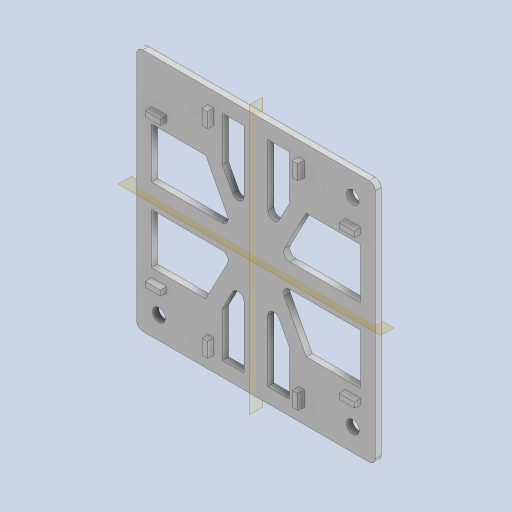
# Autodesk Inventor part: BLTouch-Leveling-Plate_V2
Saved by Autodesk Inventor 2023.2 (Build 272271000, 271)
## iProperties
Created: 2024-02-15
Part Number: BLTouch-Leveling-Plate_V2
Material: Generisch
Document SubType Name: Modeling
Designer: Nils Bade
Density: 1 g/cm^3
Appearance: Vorgabe
Description: Dummy
Auf Bestellliste: True
Author: Nils Bade
Autodesk Inventor part; units mm, degrees
ref_plane "XY Plane" through (0, 0, 0) normal (0, 0, 1) x (1, 0, 0)
sketch "S-Basis" plane through (0, 0, 0) normal (0, 0, 1) x (1, 0, 0)
  line L0 (0, 57.19) -> (0, -57.19) construction
  line L1 (-56, 0) -> (56, 0) construction
  line L2 (-40, 40.85) -> (40, 40.85)
  line L3 (40, 40.85) -> (40, -40.85)
  line L4 (40, -40.85) -> (-40, -40.85)
  line L5 (-40, -40.85) -> (-40, 40.85)
  line L6 (-40, 40.85) -> (40, -40.85) construction
  line L7 (40, 40.85) -> (-40, -40.85) construction
  line L8 (-40, 33.35) -> (40, 33.35) construction
  line L9 (-40, 13.03) -> (40, 13.03) construction
  circle A0 centre (32.5, 33.35) radius 2.15
  circle A1 centre (-32.5, -33.35) radius 2.15
  circle A2 centre (32.5, -33.35) radius 2.15
  line L10 (-40, -40.85) -> (-16.2, -40.85) construction
  line L11 (-16.2, -40.85) -> (-16.2, -25.85) construction
  line L12 (-16.2, -25.85) -> (-40, -25.85) construction
  line L13 (-40, -25.85) -> (-40, -40.85) construction
  line L14 (-40, 40.85) -> (-16.2, 40.85) construction
  line L15 (-16.2, 40.85) -> (-16.2, 25.85) construction
  line L16 (-16.2, 25.85) -> (-40, 25.85) construction
  line L17 (-40, 25.85) -> (-40, 40.85) construction
  line L18 (40, -40.85) -> (16.2, -40.85) construction
  line L19 (16.2, -40.85) -> (16.2, -25.85) construction
  line L20 (16.2, -25.85) -> (40, -25.85) construction
  line L21 (40, -25.85) -> (40, -40.85) construction
  line L22 (40, 40.85) -> (16.2, 40.85) construction
  line L23 (40, 25.85) -> (40, 40.85) construction
  line L24 (16.2, 25.85) -> (40, 25.85) construction
  line L25 (16.2, 40.85) -> (16.2, 25.85) construction
  line L26 (-16.2, -35.85) -> (-14.2, -35.85)
  line L27 (-14.2, -35.85) -> (-14.2, -30.85)
  line L28 (-14.2, -30.85) -> (-16.2, -30.85)
  line L29 (-16.2, -30.85) -> (-16.2, -35.85)
  line L30 (-35, -25.85) -> (-30, -25.85)
  line L31 (-30, -25.85) -> (-30, -23.85)
  line L32 (-30, -23.85) -> (-35, -23.85)
  line L33 (-35, -23.85) -> (-35, -25.85)
  line L34 (-16.2, 35.85) -> (-14.2, 35.85)
  line L35 (-14.2, 35.85) -> (-14.2, 30.85)
  line L36 (-14.2, 30.85) -> (-16.2, 30.85)
  line L37 (-16.2, 30.85) -> (-16.2, 35.85)
  line L38 (-35, 25.85) -> (-30, 25.85)
  line L39 (-30, 25.85) -> (-30, 23.85)
  line L40 (-30, 23.85) -> (-35, 23.85)
  line L41 (-35, 23.85) -> (-35, 25.85)
  line L42 (16.2, -35.85) -> (14.2, -35.85)
  line L43 (14.2, -35.85) -> (14.2, -30.85)
  line L44 (14.2, -30.85) -> (16.2, -30.85)
  line L45 (16.2, -30.85) -> (16.2, -35.85)
  line L46 (35, -25.85) -> (30, -25.85)
  line L47 (30, -25.85) -> (30, -23.85)
  line L48 (30, -23.85) -> (35, -23.85)
  line L49 (35, -23.85) -> (35, -25.85)
  line L50 (14.2, 30.85) -> (16.2, 30.85)
  line L51 (14.2, 35.85) -> (14.2, 30.85)
  line L52 (16.2, 35.85) -> (14.2, 35.85)
  line L53 (16.2, 30.85) -> (16.2, 35.85)
  line L54 (30, 25.85) -> (30, 23.85)
  line L55 (30, 23.85) -> (35, 23.85)
  line L56 (35, 23.85) -> (35, 25.85)
  line L57 (35, 25.85) -> (30, 25.85)
  circle A3 centre (-32.5, 33.35) radius 2.15
  point P0 (-16.2, -33.35)
  point P1 (-16.2, 33.35)
  point P2 (16.2, -33.35)
  point P3 (16.2, 33.35)
  dimension "d0" = 81.7
  dimension "d1" = 80
  dimension "d9" = 4.3
  dimension "d10" = 32.5
  dimension "d11" = 7.5
  dimension "d26" = 15
  dimension "d27" = 23.8
  dimension "d30" = 5
  dimension "d31" = 5
  dimension "d32" = 5
  dimension "d33" = 2
  dimension "d34" = 2
  constraints: 112 end point, 38 symmetric about line, 8 parallel, 6 perpendicular, 6 point on line, 4 centre point, 4 horizontal, 2 midpoint, 2 other
  measures "d0" distance of L2.end L3.end
  measures "d1" distance of L2.start L2.end
  measures "d9" diameter of A1
  measures "d10" distance from line of L0 A1.centre
  measures "d11" distance from line of L4 A1.centre
  measures "d26" distance between parallel lines of L4 L12
  measures "d27" distance between parallel lines of L5 L11
  measures "d30" distance between parallel lines of L28 L26
  measures "d31" distance between parallel lines of L31 L33
  measures "d32" distance between parallel lines of L5 L33
  measures "d33" distance between parallel lines of L12 L32
  measures "d34" distance between parallel lines of L11 L27
ref_plane "Anschlussebene-Übergang" through (-40, 13.03, 0) normal (0, 1, 0) x (1, 0, 0)
extrude "Ex-Base1" add sketch "S-Basis" against normal blind 2 contours L2 L3 L4 L5 | L29 L28 L27 L26 | L33 L32 L31 L30 | L34 L35 L36 L37 | L38 L39 L40 L41 | L42 L43 L44 L45 | L46 L47 L48 L49 | L51 L52 L53 L50 | L57 L56 L55 L54 | A3
fillet "Rundung1" radius 2 4 edges at (40, -40.85, -1) (-40, -40.85, -1) (40, 40.85, -1) (-40, 40.85, -1)
extrude "Ex-Platte-ProbeHead-Formschluss" add sketch "S-Basis" along normal blind 2 contours L29 L28 L27 L26 | L33 L32 L31 L30
chamfer "Fase-formschluss-1" distance 2 angle 5 1 edges at (-16.2, -33.35, 2) measured on face at (-16.2, -33.35, 1.5)
chamfer "Fase-formschluss-2" distance 2 angle 5 1 edges at (-32.5, -25.85, 2) measured on face at (-32.5, -25.85, 1.5)
mirror "Spiegeln1" about plane through (0, 0, 0) normal (0, 1, 0) of "Ex-Platte-ProbeHead-Formschluss", "Fase-formschluss-1", "Fase-formschluss-2"
mirror "Spiegeln2" about plane through (0, 0, 0) normal (1, 0, 0) of "Ex-Platte-ProbeHead-Formschluss", "Fase-formschluss-1", "Fase-formschluss-2", "Spiegeln1"
sketch "S-ResinSave" plane through (0, 0, 0) normal (0, 0, 1) x (1, 0, 0)
  line L0 (0, 57.19) -> (0, -57.19) construction
  line L1 (-35, -4) -> (-35, -20.85)
  line L2 (-35, -20.85) -> (-16.8473, -20.85)
  line L3 (-16.8473, -20.85) -> (-8, -4)
  line L4 (-8, -4) -> (-35, -4)
  line L5 (-11.2, -20.85) -> (-11.2, -35.85)
  line L6 (-11.2, -35.85) -> (-4, -35.85)
  line L7 (-4, -35.85) -> (-4, -7.1374)
  line L8 (-4, -7.1374) -> (-11.2, -20.85)
  line L9 (-35, -23.85) -> (-35, -25.675) construction
  line L10 (-14.2, -35.85) -> (-14.2, -30.85) construction
  line L11 (-30, -23.85) -> (-35, -23.85) construction
  line L12 (-16.025, -35.85) -> (-14.2, -35.85) construction
  line L13 (-56, 0) -> (56, 0) construction
  line L14 (-30, 23.85) -> (-35, 23.85) construction
  line L15 (35, -4) -> (35, -20.85)
  line L16 (35, -20.85) -> (16.8473, -20.85)
  line L17 (16.8473, -20.85) -> (8, -4)
  line L18 (8, -4) -> (35, -4)
  line L19 (11.2, -20.85) -> (11.2, -35.85)
  line L20 (11.2, -35.85) -> (4, -35.85)
  line L21 (4, -35.85) -> (4, -7.1374)
  line L22 (4, -7.1374) -> (11.2, -20.85)
  line L23 (-35, 4) -> (-35, 20.85)
  line L24 (-35, 20.85) -> (-16.8473, 20.85)
  line L25 (-16.8473, 20.85) -> (-8, 4)
  line L26 (-8, 4) -> (-35, 4)
  line L27 (-11.2, 20.85) -> (-11.2, 35.85)
  line L28 (-11.2, 35.85) -> (-4, 35.85)
  line L29 (-4, 35.85) -> (-4, 7.1374)
  line L30 (-4, 7.1374) -> (-11.2, 20.85)
  line L31 (35, 4) -> (35, 20.85)
  line L32 (8, 4) -> (35, 4)
  line L33 (16.8473, 20.85) -> (8, 4)
  line L34 (35, 20.85) -> (16.8473, 20.85)
  line L35 (11.2, 20.85) -> (11.2, 35.85)
  line L36 (4, 7.1374) -> (11.2, 20.85)
  line L37 (4, 35.85) -> (4, 7.1374)
  line L38 (11.2, 35.85) -> (4, 35.85)
  point P0 (0, 0)
  dimension "d74" = 4
  dimension "d75" = 3
  dimension "d76" = 3
  dimension "d77" = 5
  dimension "d78" = 4
  constraints: 64 end point, 24 symmetric about line, 4 point on line, 2 collinear, 2 parallel, 2 perpendicular, 2 vertical
  measures "d74" distance between parallel lines of L0 L7
  measures "d75" distance between parallel lines of L10 L5
  measures "d76" distance between parallel lines of L11 L2
  measures "d77" distance between parallel lines of L8 L3
  measures "d78" distance between parallel lines of L4 L13
extrude "Ex-ResinSave" cut sketch "S-ResinSave" against normal blind 2
fillet "Run-ResinSave" radius 2 8 edges at (-4, -7.1374, -1) (-8, -4, -1) (4, -7.1374, -1) (8, -4, -1) (8, 4, -1) (4, 7.1374, -1) (-4, 7.1374, -1) (-8, 4, -1)
equation "\"d10\" = d8"
equation "\"d11\" = d4"
equation "\"d8\" = 32.5"
equation "\"d4\" = 7.5"
